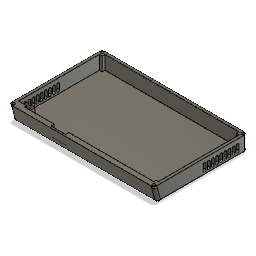
Picture Frame (Autodesk Fusion 360 design; units mm, degrees)
Autodesk Fusion 360 part; units mm, degrees
sketch "Sketch1" plane through (0, 0, 0) normal (0, 1, 0) x (1, 0, 0)
  line L0 (-60, 30) -> (204, 30)
  line L1 (204, 30) -> (204, -140)
  line L2 (204, -140) -> (-60, -140)
  line L3 (-60, -140) -> (-60, 30)
  dimension "d1" = 264
  dimension "d2" = 170
  constraint horizontal L0
  constraint vertical L1
  constraint horizontal L2
  constraint vertical L3
  measures "d1" distance of L0.start L0.end
  measures "d2" distance of L0.start L2.end
extrude "Extrude1" add sketch "Sketch1" along normal blind 30 makes body 1
sketch "Sketch2" plane through (204, 0, 0) normal (1, 0, 0) x (0, 0, -1)
  line L0 (-140, 0) -> (30, 0)
  line L1 (30, 0) -> (30, 30)
  line L2 (30, 30) -> (-140, 30)
  line L3 (-140, 30) -> (-140, 0)
  line L4 (-140, 30) -> (-114.5502, -64.9798)
  line L5 (-140, 30) -> (-41.6697, 30) construction
  line L6 (-131.9615, 0) -> (-140, 0)
  line L7 (-140, 30) -> (-140, 0)
  dimension "d6" = 75
  constraint horizontal L5
  constraint coincident L2.end L3.start
  constraint coincident L0 L6.start
  constraint coincident L4 L6.start
  constraint coincident L0.start L3.end
  measures "d6" angle of L4 L5
extrude "Extrude2" cut sketch "Sketch2" against normal blind 264 contours L0 L3 L4 L6 L7 bodies 1
sketch "Sketch3" plane through (0, 30, 0) normal (0, 1, 0) x (-1, 0, 0)
  line L0 (60, 140) -> (-204, 140)
  line L1 (-204, 140) -> (-204, -30)
  line L2 (-204, -30) -> (60, -30)
  line L3 (60, -30) -> (60, 140)
  line L4 (55, -25) -> (-199, -25)
  line L5 (-199, -25) -> (-199, 126.9615)
  line L6 (-199, 126.9615) -> (55, 126.9615)
  line L7 (55, 126.9615) -> (55, -25)
  point P0 (60, 131.9615)
  dimension "d9" = 5
  dimension "d10" = 5
  dimension "d11" = 5
  dimension "d12" = 5
  constraint horizontal L4
  constraint vertical L5
  constraint horizontal L6
  constraint vertical L7
  measures "d9" horizontal distance of L6.end P0
  measures "d10" distance of L6 P0
  measures "d11" distance of L2 L4
  measures "d12" distance of L1 L5
extrude "Extrude3" cut sketch "Sketch3" against normal blind 25 contours L4 L5 L6 L7 bodies 1
sketch "Sketch7" plane through (204, 0, 0) normal (1, 0, 0) x (0, 0, -1)
  line L0 (-140, 30) -> (-131.9615, 0)
  line L1 (-131.9615, 0) -> (30, 0)
  line L2 (30, 0) -> (30, 30)
  line L3 (30, 30) -> (-140, 30)
  line L4 (-117.5399, 20.3737) -> (-117.5395, 20.3737)
  line L5 (-117.5395, 20.3737) -> (-117.5395, 20.3317)
  line L6 (-117.5395, 10.4158) -> (-117.5399, 10.4158)
  line L7 (-112.54, 20.3491) -> (-112.5399, 10.3737)
  arc A0 (-112.54, 20.3491) -> (-117.5395, 20.3317) centre (-115.0399, 20.3737) ccw
  arc A1 (-117.5395, 10.4158) -> (-112.5399, 10.3737) centre (-115.0399, 10.3737) ccw
  line L8 (-117.5399, 20.3737) -> (-117.5399, 10.4158)
  line L9 (-110.0826, 20.3737) -> (-110.0826, 10.4158)
  line L10 (-110.0823, 10.4158) -> (-110.0826, 10.4158)
  line L11 (-110.0826, 20.3737) -> (-110.0823, 20.3737)
  arc A2 (-105.0827, 20.3491) -> (-110.0823, 20.3317) centre (-107.5826, 20.3737) ccw
  arc A3 (-110.0823, 10.4158) -> (-105.0826, 10.3737) centre (-107.5826, 10.3737) ccw
  line L12 (-105.0827, 20.3491) -> (-105.0826, 10.3737)
  line L13 (-110.0823, 20.3737) -> (-110.0823, 20.3317)
  line L14 (-102.5627, 20.405) -> (-102.5627, 10.4472)
  line L15 (-102.5623, 10.4472) -> (-102.5627, 10.4472)
  line L16 (-102.5627, 20.405) -> (-102.5623, 20.405)
  arc A4 (-97.5628, 20.3805) -> (-102.5623, 20.363) centre (-100.0627, 20.405) ccw
  arc A5 (-102.5623, 10.4472) -> (-97.5627, 10.4051) centre (-100.0627, 10.405) ccw
  line L17 (-97.5628, 20.3805) -> (-97.5627, 10.4051)
  line L18 (-102.5623, 20.405) -> (-102.5623, 20.363)
  line L19 (-80.0758, 10.5078) -> (-80.0761, 10.5078)
  line L20 (-80.0761, 20.4657) -> (-80.0761, 10.5078)
  line L21 (-87.5957, 10.4765) -> (-87.5961, 10.4765)
  line L22 (-95.053, 10.4765) -> (-95.0534, 10.4765)
  arc A6 (-90.0535, 20.4098) -> (-95.053, 20.3923) centre (-92.5534, 20.4343) ccw
  line L23 (-95.0534, 20.4343) -> (-95.0534, 10.4765)
  line L24 (-90.0535, 20.4098) -> (-90.0534, 10.4344)
  line L25 (-95.0534, 20.4343) -> (-95.053, 20.4343)
  line L26 (-87.5961, 20.4343) -> (-87.5961, 10.4765)
  line L27 (-82.5962, 20.4098) -> (-82.5961, 10.4344)
  arc A7 (-75.0763, 20.4411) -> (-80.0758, 20.4236) centre (-77.5761, 20.4657) ccw
  line L28 (-80.0761, 20.4657) -> (-80.0758, 20.4657)
  arc A8 (-80.0758, 10.5078) -> (-75.0761, 10.4657) centre (-77.5761, 10.4657) ccw
  line L29 (-80.0758, 20.4657) -> (-80.0758, 20.4236)
  line L30 (-75.0763, 20.4411) -> (-75.0761, 10.4657)
  arc A9 (-82.5962, 20.4098) -> (-87.5957, 20.3923) centre (-85.0961, 20.4343) ccw
  line L31 (-87.5961, 20.4343) -> (-87.5957, 20.4343)
  line L32 (-87.5957, 20.4343) -> (-87.5957, 20.3923)
  line L33 (-95.053, 20.4343) -> (-95.053, 20.3923)
  arc A10 (-87.5957, 10.4765) -> (-82.5961, 10.4344) centre (-85.0961, 10.4343) ccw
  arc A11 (-95.053, 10.4765) -> (-90.0534, 10.4344) centre (-92.5534, 10.4343) ccw
  line L34 (-50.0599, 20.5098) -> (-50.0599, 10.5519)
  line L35 (-30.0828, 20.5165) -> (-30.0827, 10.5411)
  line L36 (-37.6028, 20.4852) -> (-37.6026, 10.5098)
  line L37 (-42.6023, 10.5519) -> (-42.6026, 10.5519)
  line L38 (-35.0823, 10.5832) -> (-35.0827, 10.5832)
  arc A12 (-60.0893, 20.4246) -> (-65.0888, 20.4071) centre (-62.5892, 20.4491) ccw
  line L39 (-35.0823, 20.5411) -> (-35.0823, 20.4991)
  line L40 (-35.0827, 20.5411) -> (-35.0827, 10.5832)
  line L41 (-35.0827, 20.5411) -> (-35.0823, 20.5411)
  arc A13 (-30.0828, 20.5165) -> (-35.0823, 20.4991) centre (-32.5827, 20.5411) ccw
  line L42 (-45.06, 20.4852) -> (-45.0599, 10.5098)
  line L43 (-50.0599, 20.5098) -> (-50.0596, 20.5098)
  line L44 (-50.0596, 20.5098) -> (-50.0596, 20.4677)
  arc A14 (-37.6028, 20.4852) -> (-42.6023, 20.4677) centre (-40.1026, 20.5098) ccw
  arc A15 (-45.06, 20.4852) -> (-50.0596, 20.4677) centre (-47.5599, 20.5098) ccw
  line L45 (-42.6026, 20.5098) -> (-42.6023, 20.5098)
  arc A16 (-50.0596, 10.5519) -> (-45.0599, 10.5098) centre (-47.5599, 10.5098) ccw
  arc A17 (-42.6023, 10.5519) -> (-37.6026, 10.5098) centre (-40.1026, 10.5098) ccw
  line L46 (-65.0892, 20.4491) -> (-65.0888, 20.4491)
  line L47 (-65.0888, 20.4491) -> (-65.0888, 20.4071)
  arc A18 (-67.5466, 20.4246) -> (-72.5461, 20.4071) centre (-70.0465, 20.4491) ccw
  line L48 (-72.5461, 20.4491) -> (-72.5461, 20.4071)
  line L49 (-52.5694, 20.4559) -> (-52.5692, 10.4805)
  line L50 (-57.5689, 20.4805) -> (-57.5689, 20.4384)
  line L51 (-50.0596, 10.5519) -> (-50.0599, 10.5519)
  line L52 (-42.6026, 20.5098) -> (-42.6026, 10.5519)
  arc A19 (-35.0823, 10.5832) -> (-30.0827, 10.5411) centre (-32.5827, 10.5411) ccw
  line L53 (-42.6023, 20.5098) -> (-42.6023, 20.4677)
  line L54 (-72.5465, 20.4491) -> (-72.5465, 10.4913)
  arc A20 (-72.5461, 10.4913) -> (-67.5465, 10.4492) centre (-70.0465, 10.4491) ccw
  line L55 (-57.5692, 20.4805) -> (-57.5689, 20.4805)
  line L56 (-72.5465, 20.4491) -> (-72.5461, 20.4491)
  line L57 (-67.5466, 20.4246) -> (-67.5465, 10.4492)
  line L58 (-72.5461, 10.4913) -> (-72.5465, 10.4913)
  line L59 (-65.0888, 10.4913) -> (-65.0892, 10.4913)
  line L60 (-65.0892, 20.4491) -> (-65.0892, 10.4913)
  arc A21 (-65.0888, 10.4913) -> (-60.0892, 10.4492) centre (-62.5892, 10.4491) ccw
  arc A22 (-52.5694, 20.4559) -> (-57.5689, 20.4384) centre (-55.0692, 20.4805) ccw
  line L61 (-57.5692, 20.4805) -> (-57.5692, 10.5226)
  line L62 (-60.0893, 20.4246) -> (-60.0892, 10.4492)
  arc A23 (-57.5689, 10.5226) -> (-52.5692, 10.4805) centre (-55.0692, 10.4805) ccw
  line L63 (-57.5689, 10.5226) -> (-57.5692, 10.5226)
  line L64 (-5.0126, 20.4343) -> (-5.0126, 10.4765)
  line L65 (14.9645, 20.4411) -> (14.9646, 10.4657)
  line L66 (7.4445, 20.4098) -> (7.4446, 10.4344)
  line L67 (2.445, 10.4765) -> (2.4446, 10.4765)
  line L68 (9.9649, 10.5078) -> (9.9646, 10.5078)
  arc A24 (-15.042, 20.3491) -> (-20.0415, 20.3317) centre (-17.5419, 20.3737) ccw
  line L69 (9.9649, 20.4657) -> (9.9649, 20.4236)
  line L70 (9.9646, 20.4657) -> (9.9646, 10.5078)
  line L71 (9.9646, 20.4657) -> (9.9649, 20.4657)
  arc A25 (14.9645, 20.4411) -> (9.9649, 20.4236) centre (12.4646, 20.4657) ccw
  line L72 (-0.0128, 20.4098) -> (-0.0126, 10.4344)
  line L73 (-5.0126, 20.4343) -> (-5.0123, 20.4343)
  line L74 (-5.0123, 20.4343) -> (-5.0123, 20.3923)
  arc A26 (7.4445, 20.4098) -> (2.445, 20.3923) centre (4.9446, 20.4343) ccw
  arc A27 (-0.0128, 20.4098) -> (-5.0123, 20.3923) centre (-2.5126, 20.4343) ccw
  line L75 (2.4446, 20.4343) -> (2.445, 20.4343)
  arc A28 (-5.0123, 10.4765) -> (-0.0126, 10.4344) centre (-2.5126, 10.4343) ccw
  arc A29 (2.445, 10.4765) -> (7.4446, 10.4344) centre (4.9446, 10.4343) ccw
  line L76 (-20.0419, 20.3737) -> (-20.0415, 20.3737)
  line L77 (-20.0415, 20.3737) -> (-20.0415, 20.3317)
  arc A30 (-22.4993, 20.3491) -> (-27.4988, 20.3317) centre (-24.9992, 20.3737) ccw
  line L78 (-27.4988, 20.3737) -> (-27.4988, 20.3317)
  line L79 (-7.5221, 20.3805) -> (-7.522, 10.4051)
  line L80 (-12.5216, 20.405) -> (-12.5216, 20.363)
  line L81 (-5.0123, 10.4765) -> (-5.0126, 10.4765)
  line L82 (2.4446, 20.4343) -> (2.4446, 10.4765)
  arc A31 (9.9649, 10.5078) -> (14.9646, 10.4657) centre (12.4646, 10.4657) ccw
  line L83 (2.445, 20.4343) -> (2.445, 20.3923)
  line L84 (-27.4992, 20.3737) -> (-27.4992, 10.4158)
  arc A32 (-27.4988, 10.4158) -> (-22.4992, 10.3737) centre (-24.9992, 10.3737) ccw
  line L85 (-12.522, 20.405) -> (-12.5216, 20.405)
  line L86 (-27.4992, 20.3737) -> (-27.4988, 20.3737)
  line L87 (-22.4993, 20.3491) -> (-22.4992, 10.3737)
  line L88 (-27.4988, 10.4158) -> (-27.4992, 10.4158)
  line L89 (-20.0415, 10.4158) -> (-20.0419, 10.4158)
  line L90 (-20.0419, 20.3737) -> (-20.0419, 10.4158)
  arc A33 (-20.0415, 10.4158) -> (-15.0419, 10.3737) centre (-17.5419, 10.3737) ccw
  arc A34 (-7.5221, 20.3805) -> (-12.5216, 20.363) centre (-10.022, 20.405) ccw
  line L91 (-12.522, 20.405) -> (-12.522, 10.4472)
  line L92 (-15.042, 20.3491) -> (-15.0419, 10.3737)
  arc A35 (-12.5216, 10.4472) -> (-7.522, 10.4051) centre (-10.022, 10.405) ccw
  line L93 (-12.5216, 10.4472) -> (-12.522, 10.4472)
  dimension "d43" = 5
  dimension "d44" = 5
  dimension "d45" = 5
  dimension "d46" = 5
  dimension "d47" = 5
  dimension "d48" = 5
  dimension "d49" = 5
  dimension "d50" = 5
  dimension "d51" = 5
  dimension "d52" = 5
  dimension "d53" = 5
  dimension "d54" = 5
  dimension "d55" = 5
  dimension "d56" = 5
  dimension "d57" = 5
  dimension "d58" = 5
  dimension "d59" = 5
  dimension "d60" = 5
  dimension "d61" = 5
  dimension "d62" = 5
  dimension "d63" = 5
  dimension "d64" = 5
  dimension "d65" = 5
  dimension "d66" = 5
  dimension "d67" = 5
  dimension "d68" = 5
  dimension "d69" = 5
  dimension "d70" = 5
  dimension "d71" = 5
  dimension "d72" = 5
  dimension "d73" = 5
  dimension "d74" = 5
  dimension "d75" = 5
  dimension "d76" = 5
  dimension "d77" = 5
  dimension "d78" = 5
  constraint horizontal L4
  constraint vertical L5
  constraint horizontal L6
  constraint coincident L4.start A0
  constraint tangent L7 A1
  constraint perpendicular L6 L8
  constraint horizontal L11
  constraint vertical L13
  constraint horizontal L10
  constraint coincident L9.start A2
  constraint tangent A3 L12
  constraint perpendicular L9 L10
  constraint horizontal L16
  constraint vertical L18
  constraint horizontal L15
  constraint coincident L14.start A4
  constraint tangent A5 L17
  constraint perpendicular L14 L15
  constraint horizontal L25
  constraint vertical L33
  constraint horizontal L22
  constraint coincident L23.start A6
  constraint tangent L24 A11
  constraint perpendicular L22 L23
  constraint horizontal L31
  constraint vertical L32
  constraint horizontal L21
  constraint coincident L26.start A9
  constraint tangent L27 A10
  constraint perpendicular L21 L26
  constraint horizontal L28
  constraint vertical L29
  constraint horizontal L19
  constraint coincident L20.start A7
  constraint tangent A8 L30
  constraint perpendicular L19 L20
  constraint horizontal L56
  constraint vertical L48
  constraint horizontal L58
  constraint coincident L54.start A18
  constraint tangent A20 L57
  constraint perpendicular L54 L58
  constraint horizontal L46
  constraint vertical L47
  constraint horizontal L59
  constraint coincident L46.start A12
  constraint tangent A21 L62
  constraint perpendicular L59 L60
  constraint horizontal L55
  constraint vertical L50
  constraint horizontal L63
  constraint coincident L55.start A22
  constraint tangent L49 A23
  constraint perpendicular L61 L63
  constraint horizontal L43
  constraint vertical L44
  constraint horizontal L51
  constraint coincident L34.start A15
  constraint tangent L42 A16
  constraint perpendicular L34 L51
  constraint horizontal L45
  constraint vertical L53
  constraint horizontal L37
  constraint coincident L45.start A14
  constraint tangent L36 A17
  constraint perpendicular L37 L52
  constraint horizontal L41
  constraint vertical L39
  constraint horizontal L38
  constraint coincident L40.start A13
  constraint tangent L35 A19
  constraint perpendicular L38 L40
  constraint horizontal L86
  constraint vertical L78
  constraint horizontal L88
  constraint coincident L84.start A30
  constraint tangent A32 L87
  constraint perpendicular L84 L88
  constraint horizontal L76
  constraint vertical L77
  constraint horizontal L89
  constraint coincident L76.start A24
  constraint tangent A33 L92
  constraint perpendicular L89 L90
  constraint horizontal L85
  constraint vertical L80
  constraint horizontal L93
  constraint coincident L85.start A34
  constraint tangent L79 A35
  constraint perpendicular L91 L93
  constraint horizontal L73
  constraint vertical L74
  constraint horizontal L81
  constraint coincident L64.start A27
  constraint tangent L72 A28
  constraint perpendicular L64 L81
  constraint horizontal L75
  constraint vertical L83
  constraint horizontal L67
  constraint coincident L75.start A26
  constraint tangent L66 A29
  constraint perpendicular L67 L82
  constraint horizontal L71
  constraint vertical L69
  constraint horizontal L68
  constraint coincident L70.start A25
  constraint tangent L65 A31
  constraint perpendicular L68 L70
  measures "d43" diameter of A0
  measures "d44" diameter of A1
  measures "d45" diameter of A2
  measures "d46" diameter of A3
  measures "d47" diameter of A4
  measures "d48" diameter of A5
  measures "d49" diameter of A6
  measures "d50" diameter of A11
  measures "d51" diameter of A9
  measures "d52" diameter of A10
  measures "d53" diameter of A7
  measures "d54" diameter of A8
  measures "d55" diameter of A18
  measures "d56" diameter of A20
  measures "d57" diameter of A12
  measures "d58" diameter of A21
  measures "d59" diameter of A22
  measures "d60" diameter of A23
  measures "d61" diameter of A15
  measures "d62" diameter of A16
  measures "d63" diameter of A14
  measures "d64" diameter of A17
  measures "d65" diameter of A13
  measures "d66" diameter of A19
  measures "d67" diameter of A30
  measures "d68" diameter of A32
  measures "d69" diameter of A24
  measures "d70" diameter of A33
  measures "d71" diameter of A34
  measures "d72" diameter of A35
  measures "d73" diameter of A27
  measures "d74" diameter of A28
  measures "d75" diameter of A26
  measures "d76" diameter of A29
  measures "d77" diameter of A25
  measures "d78" diameter of A31
extrude "Extrude11" cut sketch "Sketch7" against normal blind 270 contours L5 L7 A0 A1 L8 | L9 A2 A3 L12 L13 | L14 A4 A5 L17 L18 | L20 A7 A8 L29 L30 | A6 L23 L24 L33 A11 | L26 L27 A9 L32 A10 | L34 L42 L44 A15 A16 | L35 L39 L40 A13 A19 | L36 A14 A17 L52 L53 | A12 L47 L60 A21 L62 | A18 L48 L54 A20 L57 | L49 L50 A22 L61 A23 | L64 L72 L74 A27 A28 | L65 L69 L70 A25 A31 | L66 A26 A29 L82 L83 | A24 L77 L90 A33 L92 | A30 L78 L84 A32 L87 | L79 L80 A34 L91 A35 bodies 1
sketch "Sketch8" plane through (0, 5, 0) normal (0, 1, 0) x (-1, 0, 0)
  line L0 (55, 126.9615) -> (-199, 126.9615)
  line L1 (-199, 126.9615) -> (-199, -25)
  line L2 (-199, -25) -> (55, -25)
  line L3 (55, -25) -> (55, 126.9615)
  line L4 (55, 126.9615) -> (40, 126.9615)
  line L5 (40, 126.9615) -> (40, 111.9615)
  line L6 (40, 111.9615) -> (55, 111.9615)
  line L7 (55, 111.9615) -> (55, 126.9615)
  dimension "d81" = 15
  dimension "d82" = 15
  constraint horizontal L4
  constraint vertical L5
  constraint horizontal L6
  constraint vertical L7
  constraint coincident L0.start L3.end
  measures "d81" distance of L0.start L4.end
  measures "d82" distance of L0.start L6.end
extrude "Extrude12" add sketch "Sketch8" along normal blind 17 separate body contours L0 L3 L4 L5 L6 L7 makes body 2
sketch "Sketch9" plane through (0, 22, 0) normal (0, 1, 0) x (-1, 0, 0)
  line L0 (55, 111.9615) -> (55, 126.9615)
  line L1 (55, 126.9615) -> (40, 126.9615)
  line L2 (40, 126.9615) -> (40, 111.9615)
  line L3 (40, 111.9615) -> (55, 111.9615)
  circle A0 centre (47.4433, 119.4498) radius 5.5
  dimension "d85" = 11
  measures "d85" diameter of A0
extrude "Extrude13" cut sketch "Sketch9" against normal blind 43 contours A0 bodies 1 2
sketch "Sketch10" plane through (0, 5, 0) normal (0, 1, 0) x (-1, 0, 0)
  circle A0 centre (47.4433, 119.4498) radius 5.5
  line L0 (55, 126.9615) -> (-199, 126.9615)
  line L1 (-199, 126.9615) -> (-199, -25)
  line L2 (-199, -25) -> (55, -25)
  line L3 (55, -25) -> (55, 126.9615)
sketch "Sketch11" plane through (0, 5, 0) normal (0, 1, 0) x (-1, 0, 0)
  line L0 (39.9163, 111.9948) -> (54.9163, 111.9948)
  line L1 (54.9163, 111.9948) -> (54.9163, 126.9948)
  line L2 (54.9163, 126.9948) -> (39.9163, 126.9948)
  line L3 (39.9163, 126.9948) -> (39.9163, 111.9948)
  circle A0 centre (47.5, 119.5) radius 5.5
  dimension "d88" = 15
  dimension "d89" = 15
  dimension "d90" = 11
  constraint horizontal L0
  constraint vertical L1
  constraint horizontal L2
  constraint vertical L3
  measures "d88" distance of L0 L2
  measures "d89" distance of L1 L3
  measures "d90" diameter of A0
extrude "Extrude1'" add sketch "Sketch11" along normal blind 15 separate body makes body 3 in component "Component"
sketch "Sketch15" plane through (0, 30, 0) normal (0, 1, 0) x (-1, 0, 0)
  line L0 (-199, -25) -> (-199, 126.9615)
  line L1 (-199, 126.9615) -> (55, 126.9615)
  line L2 (55, 126.9615) -> (55, -25)
  line L3 (55, -25) -> (-199, -25)
  line L4 (60, 140) -> (-204, 140)
  line L5 (-204, 140) -> (-204, -30)
  line L6 (-204, -30) -> (60, -30)
  line L7 (60, -30) -> (60, 140)
  line L8 (60, -22.7198) -> (55, -22.7198)
  line L9 (55, -22.7198) -> (55, 50.7625)
  line L10 (55, 50.7625) -> (60, 50.7625)
  line L11 (60, 50.7625) -> (60, -22.7198)
  constraint horizontal L8
  constraint vertical L9
  constraint horizontal L10
  constraint vertical L11
  constraint coincident L2 L9.end
  constraint coincident L7 L8.start
extrude "Extrude15" add sketch "Sketch15" against normal blind 30 contours L2 L7 L8 L9 L10 L11 bodies 1
sketch "Sketch16" plane through (0, 30, 0) normal (0, 1, 0) x (-1, 0, 0)
  line L0 (-204, 140) -> (-204, -30)
  line L1 (-204, -30) -> (60, -30)
  line L2 (60, -30) -> (60, 140)
  line L3 (60, 140) -> (-204, 140)
  line L4 (55, 126.9615) -> (55, -25)
  line L5 (55, -25) -> (-199, -25)
  line L6 (-199, -25) -> (-199, 126.9615)
  line L7 (-199, 126.9615) -> (55, 126.9615)
  line L8 (-199, 51.2067) -> (-204, 51.2067)
  line L9 (-204, 51.2067) -> (-204, 121.8184)
  line L10 (-204, 121.8184) -> (-199, 121.8184)
  line L11 (-199, 121.8184) -> (-199, 51.2067)
  constraint horizontal L8
  constraint vertical L9
  constraint horizontal L10
  constraint vertical L11
  constraint coincident L0 L9.end
extrude "Extrude16" add sketch "Sketch16" against normal blind 27 contours L0 L6 L8 L9 L10 L11 bodies 1
sketch "Sketch17" plane through (0, 30, 0) normal (0, 1, 0) x (-1, 0, 0)
  line L0 (-199, -25) -> (-199, 126.9615)
  line L1 (-199, 126.9615) -> (55, 126.9615)
  line L2 (55, 126.9615) -> (55, -25)
  line L3 (55, -25) -> (-199, -25)
  line L4 (-204, 140) -> (-204, -30)
  line L5 (-204, -30) -> (60, -30)
  line L6 (60, -30) -> (60, 140)
  line L7 (60, 140) -> (-204, 140)
  line L8 (-14, 126.9615) -> (-40, 126.9615)
  line L9 (-40, 126.9615) -> (-40, 130.9615)
  line L10 (-40, 130.9615) -> (-14, 130.9615)
  line L11 (-14, 130.9615) -> (-14, 126.9615)
  line L12 (60, 140) -> (60, -30)
  dimension "d107" = 100
  dimension "d108" = 74
  dimension "d109" = 4
  constraint horizontal L8
  constraint vertical L9
  constraint horizontal L10
  constraint vertical L11
  constraint coincident L1 L8.start
  measures "d107" distance of L9 L12
  measures "d108" distance of L11 L12
  measures "d109" distance of L8 L10
extrude "Extrude17" cut sketch "Sketch17" against normal blind 25 contours L1 L8 L9 L10 L11 bodies 1
fillet "Fillet5" radius 3 1 edges at (27, 30, 130.9615) on bodies 1
sketch "Sketch18" plane through (0, 5, 0) normal (0, 1, 0) x (-1, 0, 0)
  circle A0 centre (47.4433, 119.4498) radius 5.5
  line L0 (-40, 126.9615) -> (-199, 126.9615)
  line L1 (-199, 126.9615) -> (-199, -25)
  line L2 (-199, -25) -> (55, -25)
  line L3 (55, -25) -> (55, 126.9615)
  line L4 (55, 126.9615) -> (-14, 126.9615)
  line L5 (-14, 126.9615) -> (-14, 130.9615)
  line L6 (-14, 130.9615) -> (-40, 130.9615)
  line L7 (-40, 130.9615) -> (-40, 126.9615)
  line L8 (50, -25) -> (55, -25)
  line L9 (55, -25) -> (55, -20)
  line L10 (55, -20) -> (50, -20)
  line L11 (50, -20) -> (50, -25)
  line L12 (-199, -25) -> (-194, -25)
  line L13 (-194, -25) -> (-194, -20)
  line L14 (-194, -20) -> (-199, -20)
  line L15 (-199, -20) -> (-199, -25)
  dimension "d114" = 5
  dimension "d115" = 5
  dimension "d116" = 5
  dimension "d117" = 5
  constraint horizontal L8
  constraint vertical L9
  constraint horizontal L10
  constraint vertical L11
  constraint coincident L3 L9.end
  constraint coincident L2 L8.start
  constraint horizontal L12
  constraint vertical L13
  constraint horizontal L14
  constraint vertical L15
  constraint coincident L1.end L2.start
  measures "d114" distance of L9 L11
  measures "d115" distance of L8 L10
  measures "d116" distance of L1.end L12.end
  measures "d117" distance of L1.end L14.end
extrude "Extrude18" add sketch "Sketch18" along normal blind 25 contours L1 L2 L12 L13 L14 L15 | L2 L3 L8 L9 L10 L11 bodies 1
sketch "Sketch19" plane through (0, 30, 0) normal (0, 1, 0) x (-1, 0, 0)
  line L0 (-14, 133.9615) -> (-14, 126.9615)
  line L1 (-14, 126.9615) -> (55, 126.9615)
  line L2 (55, 126.9615) -> (55, -20)
  line L3 (55, -20) -> (50, -20)
  line L4 (50, -20) -> (50, -25)
  line L5 (50, -25) -> (-194, -25)
  line L6 (-194, -25) -> (-194, -20)
  line L7 (-194, -20) -> (-199, -20)
  line L8 (-199, -20) -> (-199, 126.9615)
  line L9 (-199, 126.9615) -> (-40, 126.9615)
  line L10 (-40, 126.9615) -> (-40, 133.9615)
  line L11 (-40, 133.9615) -> (-14, 133.9615)
  line L12 (-204, 140) -> (-204, -30)
  line L13 (-204, -30) -> (60, -30)
  line L14 (60, -30) -> (60, 140)
  line L15 (60, 140) -> (-204, 140)
  circle A0 centre (-200.1656, -25.9) radius 2.75
  line L16 (-197.2656, -30) -> (-204.2656, -30)
  line L17 (-204.2656, -30) -> (-204.2656, -23)
  line L18 (-204.2656, -23) -> (-197.2656, -23)
  line L19 (-197.2656, -23) -> (-197.2656, -30)
  dimension "d120" = 5.5
  dimension "d121" = 7
  dimension "d122" = 7
  dimension "d123" = 2.9
  dimension "d124" = 2.9
  constraint horizontal L16
  constraint vertical L17
  constraint horizontal L18
  constraint vertical L19
  constraint coincident L13 L16.start
  measures "d120" diameter of A0
  measures "d121" distance of L16.start L16.end
  measures "d122" distance of L16.start L18.end
  measures "d123" distance of A0.centre L19
  measures "d124" distance of A0.centre L18
sketch "Sketch14" plane through (0, 30, 0) normal (0, 1, 0) x (-1, 0, 0)
  line L0 (60, 140) -> (-204, 140)
  line L1 (-204, 140) -> (-204, -30)
  line L2 (-204, -30) -> (60, -30)
  line L3 (60, -30) -> (60, 140)
  line L4 (-199, -20) -> (-199, 126.9615)
  line L5 (-14, 126.9615) -> (55, 126.9615)
  line L6 (55, 126.9615) -> (55, -20)
  line L7 (50, -25) -> (-194, -25)
  line L8 (60, -30) -> (57.1, -30)
  line L9 (60, -30) -> (60, -27.1)
  line L10 (-14, 133.9615) -> (-14, 126.9615)
  line L11 (55, -20) -> (50, -20)
  line L12 (50, -20) -> (50, -25)
  line L13 (-194, -25) -> (-194, -20)
  line L14 (-194, -20) -> (-199, -20)
  line L15 (-199, 126.9615) -> (-40, 126.9615)
  line L16 (-40, 126.9615) -> (-40, 133.9615)
  line L17 (-40, 133.9615) -> (-14, 133.9615)
  constraint horizontal L8
  constraint perpendicular L8 L9
fillet "Fillet6" radius 5 8 edges at (-60, 15, -30) (-60, 15, 135.9808) (204, 15, -30) (204, 15, 135.9808) (204, 0, 50.9808) (72, 0, 131.9615) (72, 0, -30) (-60, 0, 50.9808) on bodies 1
sketch "Sketch20" plane through (0, 30, 0) normal (0, 1, 0) x (-1, 0, 0)
  arc A0 (-204, -25) -> (-199, -30) centre (-199, -25) ccw
  line L0 (-199, -30) -> (55, -30)
  arc A1 (55, -30) -> (60, -25) centre (55, -25) ccw
  line L1 (60, -25) -> (60, 134.8236)
  ellipse E0 centre (55, 134.8236) end of major axis (55, 140) minor radius 5 (60, 134.8236) -> (55, 140) ccw
  line L2 (55, 140) -> (-199, 140)
  ellipse E1 centre (-199, 134.8236) end of major axis (-199, 140) minor radius 5 (-199, 140) -> (-204, 134.8236) ccw
  line L3 (-204, 134.8236) -> (-204, -25)
  line L4 (-14, 133.9615) -> (-14, 126.9615)
  line L5 (-14, 126.9615) -> (55, 126.9615)
  line L6 (55, 126.9615) -> (55, -20)
  line L7 (55, -20) -> (50, -20)
  line L8 (50, -20) -> (50, -25)
  line L9 (50, -25) -> (-194, -25)
  line L10 (-194, -25) -> (-194, -20)
  line L11 (-194, -20) -> (-199, -20)
  line L12 (-199, -20) -> (-199, 126.9615)
  line L13 (-199, 126.9615) -> (-40, 126.9615)
  line L14 (-40, 126.9615) -> (-40, 133.9615)
  line L15 (-40, 133.9615) -> (-14, 133.9615)
  line L16 (53, -30) -> (53, -23)
  line L17 (53, -23) -> (60, -23)
  line L18 (60, -23) -> (60, -30)
  dimension "d128" = 7
  dimension "d129" = 7
  constraint vertical L16
  constraint horizontal L17
  constraint vertical L18
  measures "d128" distance of L18.end L16.start
  measures "d129" distance of L18.end L17.end
sketch "Sketch21" plane through (0, 30, 0) normal (0, 1, 0) x (-1, 0, 0)
  arc A0 (-204, -25) -> (-199, -30) centre (-199, -25) ccw
  line L0 (-199, -30) -> (55, -30)
  arc A1 (55, -30) -> (60, -25) centre (55, -25) ccw
  line L1 (60, -25) -> (60, 134.8236)
  ellipse E0 centre (55, 134.8236) end of major axis (55, 140) minor radius 5 (60, 134.8236) -> (55, 140) ccw
  line L2 (55, 140) -> (-199, 140)
  ellipse E1 centre (-199, 134.8236) end of major axis (-199, 140) minor radius 5 (-199, 140) -> (-204, 134.8236) ccw
  line L3 (-204, 134.8236) -> (-204, -25)
  line L4 (-14, 133.9615) -> (-14, 126.9615)
  line L5 (-14, 126.9615) -> (55, 126.9615)
  line L6 (55, 126.9615) -> (55, -20)
  line L7 (55, -20) -> (50, -20)
  line L8 (50, -20) -> (50, -25)
  line L9 (50, -25) -> (-194, -25)
  line L10 (-194, -25) -> (-194, -20)
  line L11 (-194, -20) -> (-199, -20)
  line L12 (-199, -20) -> (-199, 126.9615)
  line L13 (-199, 126.9615) -> (-40, 126.9615)
  line L14 (-40, 126.9615) -> (-40, 133.9615)
  line L15 (-40, 133.9615) -> (-14, 133.9615)
extrude "Extrude19" cut sketch "Sketch19" against normal blind 4.5 contours A0 bodies 1
sketch "Sketch22" plane through (0, 30, 0) normal (0, 1, 0) x (-1, 0, 0)
sketch "Sketch23" plane through (0, 30, 0) normal (0, 1, 0) x (-1, 0, 0)
  circle A0 centre (55.8901, -25.8454) radius 2.75
  dimension "d136" = 5.5
  measures "d136" diameter of A0
extrude "Extrude20" cut sketch "Sketch23" against normal blind 4.5 bodies 1
sketch "Sketch24" plane through (0, 30, 0) normal (0, 1, 0) x (-1, 0, 0)
  circle A0 centre (55.8525, 135.8512) radius 2.75
  line L0 (60, 140) -> (53, 140)
  line L1 (53, 140) -> (53, 133)
  line L2 (53, 133) -> (60, 133)
  line L3 (60, 133) -> (60, 140)
  dimension "d139" = 5.5
  dimension "d140" = 7
  dimension "d141" = 7
  constraint horizontal L0
  constraint vertical L1
  constraint horizontal L2
  constraint vertical L3
  measures "d139" diameter of A0
  measures "d140" distance of L0.start L0.end
  measures "d141" distance of L0.start L2.end
extrude "Extrude21" cut sketch "Sketch24" against normal blind 4.5 contours A0 bodies 1
sketch "Sketch25" plane through (0, 30, 0) normal (0, 1, 0) x (-1, 0, 0)
  line L0 (-204, 140) -> (-197, 140)
  line L1 (-197, 140) -> (-197, 133)
  line L2 (-197, 133) -> (-204, 133)
  line L3 (-204, 133) -> (-204, 140)
  circle A0 centre (-199.8509, 135.8305) radius 2.75
  dimension "d144" = 7
  dimension "d145" = 7
  dimension "d146" = 5.5
  constraint horizontal L0
  constraint vertical L1
  constraint horizontal L2
  constraint vertical L3
  measures "d144" distance of L0.start L0.end
  measures "d145" distance of L0.start L2.end
  measures "d146" diameter of A0
extrude "Extrude22" cut sketch "Sketch25" against normal blind 4.5 contours A0 bodies 1
sketch "Sketch26" plane through (0, 30, 0) normal (0, 1, 0) x (-1, 0, 0)
  circle A0 centre (-199.8509, 135.8305) radius 2.75
  circle A1 centre (55.8525, 135.8512) radius 2.75
  circle A2 centre (55.8901, -25.8454) radius 2.75
  circle A3 centre (-200.1656, -25.9) radius 2.75
  arc A4 (-204, -25) -> (-199, -30) centre (-199, -25) ccw
  line L0 (-199, -30) -> (55, -30)
  arc A5 (55, -30) -> (60, -25) centre (55, -25) ccw
  line L1 (60, -25) -> (60, 134.8236)
  ellipse E0 centre (55, 134.8236) end of major axis (55, 140) minor radius 5 (60, 134.8236) -> (55, 140) ccw
  line L2 (55, 140) -> (-199, 140)
  ellipse E1 centre (-199, 134.8236) end of major axis (-199, 140) minor radius 5 (-199, 140) -> (-204, 134.8236) ccw
  line L3 (-204, 134.8236) -> (-204, -25)
  line L4 (-14, 133.9615) -> (-14, 126.9615)
  line L5 (-14, 126.9615) -> (55, 126.9615)
  line L6 (55, 126.9615) -> (55, -20)
  line L7 (55, -20) -> (50, -20)
  line L8 (50, -20) -> (50, -25)
  line L9 (50, -25) -> (-194, -25)
  line L10 (-194, -25) -> (-194, -20)
  line L11 (-194, -20) -> (-199, -20)
  line L12 (-199, -20) -> (-199, 126.9615)
  line L13 (-199, 126.9615) -> (-40, 126.9615)
  line L14 (-40, 126.9615) -> (-40, 133.9615)
  line L15 (-40, 133.9615) -> (-14, 133.9615)
  line L16 (-14, 126.9615) -> (40, 126.9615)
  line L17 (40, 126.9615) -> (40, 131)
  line L18 (40, 131) -> (-14, 131)
  line L19 (-14, 131) -> (-14, 126.9615)
  line L20 (-14, 131) -> (-40, 131)
  line L21 (-40, 131) -> (-40, 133.9615)
  line L22 (-40, 133.9615) -> (-14, 133.9615)
  line L23 (-14, 133.9615) -> (-14, 131)
  line L24 (-40, 131) -> (-195.0879, 131)
  line L25 (-195.0879, 131) -> (-195.0879, 126.9615)
  line L26 (-195.0879, 126.9615) -> (-40, 126.9615)
  line L27 (-40, 126.9615) -> (-40, 131)
  constraint horizontal L16
  constraint vertical L17
  constraint horizontal L18
  constraint vertical L19
  constraint coincident L4.end L5.start
  constraint horizontal L20
  constraint vertical L21
  constraint horizontal L22
  constraint vertical L23
  constraint coincident L14.end L15.start
  constraint horizontal L24
  constraint vertical L25
  constraint horizontal L26
  constraint vertical L27
  constraint coincident L13 L25.end
extrude "Extrude23" cut sketch "Sketch26" against normal blind 25 contours L4 L5 L16 L17 L18 L19 | L13 L14 L24 L25 L26 L27 bodies 1
extrude "Extrude2'" cut sketch "Sketch26" against normal blind 25 contours L4 L5 L16 L17 L18 L19 | L13 L14 L24 L25 L26 L27 sketch seen with x (1, 0, 0) y (0, 1, 0) z (0, 0, 1) at (0.0837, 0, -0.0046) bodies 3 in component "Component"
sketch "Sketch27" plane through (0, 30, 0) normal (0, 1, 0) x (-1, 0, 0)
  line L0 (40, 131) -> (40, 126.9615)
  line L1 (40, 126.9615) -> (55, 126.9615)
  line L2 (55, 126.9615) -> (55, -20)
  line L3 (55, -20) -> (50, -20)
  line L4 (50, -20) -> (50, -25)
  line L5 (50, -25) -> (-194, -25)
  line L6 (-194, -25) -> (-194, -20)
  line L7 (-194, -20) -> (-199, -20)
  line L8 (-199, -20) -> (-199, 126.9615)
  line L9 (-199, 126.9615) -> (-195.0879, 126.9615)
  line L10 (-195.0879, 126.9615) -> (-195.0879, 131)
  line L11 (-195.0879, 131) -> (-40, 131)
  line L12 (-40, 131) -> (-40, 133.9615)
  line L13 (-40, 133.9615) -> (-14, 133.9615)
  line L14 (-14, 133.9615) -> (-14, 131)
  line L15 (-14, 131) -> (40, 131)
  circle A0 centre (-199.8509, 135.8305) radius 2.75
  circle A1 centre (55.8525, 135.8512) radius 2.75
  circle A2 centre (55.8901, -25.8454) radius 2.75
  circle A3 centre (-200.1656, -25.9) radius 2.75
  arc A4 (-204, -25) -> (-199, -30) centre (-199, -25) ccw
  line L16 (-199, -30) -> (55, -30)
  arc A5 (55, -30) -> (60, -25) centre (55, -25) ccw
  line L17 (60, -25) -> (60, 134.8236)
  ellipse E0 centre (55, 134.8236) end of major axis (55, 140) minor radius 5 (60, 134.8236) -> (55, 140) ccw
  line L18 (55, 140) -> (-199, 140)
  ellipse E1 centre (-199, 134.8236) end of major axis (-199, 140) minor radius 5 (-199, 140) -> (-204, 134.8236) ccw
  line L19 (-204, 134.8236) -> (-204, -25)
  line L20 (-14, 131) -> (-40, 131)
  line L21 (-40, 131) -> (-40, 133.9615)
  line L22 (-40, 133.9615) -> (-14, 133.9615)
  line L23 (-14, 133.9615) -> (-14, 131)
  line L24 (-14, 131.3774) -> (-39.9869, 131.3774)
  line L25 (-39.9869, 131.3774) -> (-39.9869, 129.5624)
  line L26 (-39.9869, 129.5624) -> (-14, 129.5624)
  line L27 (-14, 129.5624) -> (-14, 131.3774)
  constraint horizontal L20
  constraint vertical L21
  constraint horizontal L22
  constraint vertical L23
  constraint coincident L12.end L13.start
  constraint coincident L14.end L15.start
  constraint horizontal L24
  constraint vertical L25
  constraint horizontal L26
  constraint vertical L27
  constraint coincident L14 L24.start
extrude "Extrude25" cut sketch "Sketch27" against normal blind 25 contours L20 L25 L26 L27 bodies 1
extrude "Extrude24" cut sketch "Sketch27" against normal blind 19 contours L14 L20 L23 L24 L25 L27 | L12 L13 L14 L20 L21 L22 L23 L24 L25 bodies 1
fillet "Fillet7" radius 3 1 edges at (27, 30, 133.9615) on bodies 1
fillet "Fillet8" radius 3 1 edges at (26.9934, 11, 131) on bodies 1
component "Component" placed x (1, 0, 0) y (0, 1, 0) z (0, 0, 1) at (-0.0837, 0, 0.0046)
hidden bodies 2
equation "d83 = 22 mm - 5 mm"
